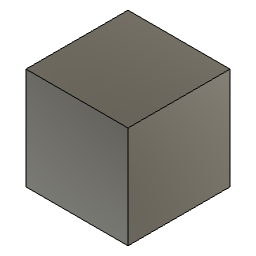
cold_shroud v4 (Autodesk Fusion 360 design; units mm, degrees)
Autodesk Fusion 360 part; units mm, degrees
sketch "Sketch9" plane through (0, 0, 0) normal (0, 0, 1) x (1, 0, 0)
  line L0 (-137.7795, 113.4984) -> (116.2205, 113.4984)
  line L1 (-137.7795, 113.4984) -> (-137.7795, -140.5016)
  line L2 (-137.7795, -140.5016) -> (116.2205, -140.5016)
  line L3 (116.2205, 113.4984) -> (116.2205, -140.5016)
  constraint horizontal L0
  constraint perpendicular L0 L1
  constraint perpendicular L1 L2
extrude "Extrude2" add sketch "Sketch9" along normal blind 254
shell "Shell2" thickness 25.4 removed faces 1 at (-53.1129, -55.835, 0)
